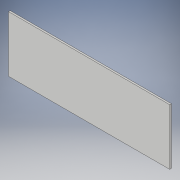
# Autodesk Inventor part: 20 bakje tussenstukje
Saved by Autodesk Inventor 2019 (Build 230136000, 136)
## iProperties
Created: 2021-01-12
Part Number: 20 bakje tussenstukje
Material: Generic
Document SubType Name: Sheet Metal
Designer: semboonen
Density: 1 g/cm^3
Sheet Metal Rule: Default_mm
Appearance: Default
Author: semboonen
Autodesk Inventor part; units mm, degrees
ref_plane "YZ Plane" through (0, 0, 0) normal (1, 0, 0) x (0, 1, 0)
ref_plane "XZ Plane" through (0, 0, 0) normal (0, 1, 0) x (-1, 0, 0)
ref_plane "XY Plane" through (0, 0, 0) normal (0, 0, 1) x (1, 0, 0)
sketch "Sketch1" plane through (0, 0, 0) normal (0, 0, 1) x (1, 0, 0)
  line L0 (-22.9, -7.95) -> (22.9, -7.95)
  line L1 (22.9, -7.95) -> (22.9, 7.95)
  line L2 (22.9, 7.95) -> (-22.9, 7.95)
  line L3 (-22.9, 7.95) -> (-22.9, -7.95)
  line L4 (-22.9, -7.95) -> (22.9, 7.95) construction
  line L5 (22.9, -7.95) -> (-22.9, 7.95) construction
  point P0 (0, 0)
  dimension "d0" = 45.8
  dimension "d1" = 15.9
  measures "d0" distance of L2.end L1.end
  measures "d1" distance of L1.end L0.end
extrude "Plate1" add sketch "Sketch1" along normal blind 0.5
equation "\"d2\" = Thickness"
equation "\"BendRadius\" = Thickness"
equation "\"BendReliefWidth\" = Thickness"
equation "\"BendReliefDepth\" = 0.5 * Thickness"
equation "\"CornerReliefSize\" = 4 * Thickness"
equation "\"MinimumRemnant\" = 2 * Thickness"
equation "\"TransitionRadius\" = BendRadius"
equation "\"JacobiRadiusSize\" = BendRadius"
equation "\"GapSize\" = Thickness"
equation "\"Thickness\" = 0.5"
body "Solid1"
